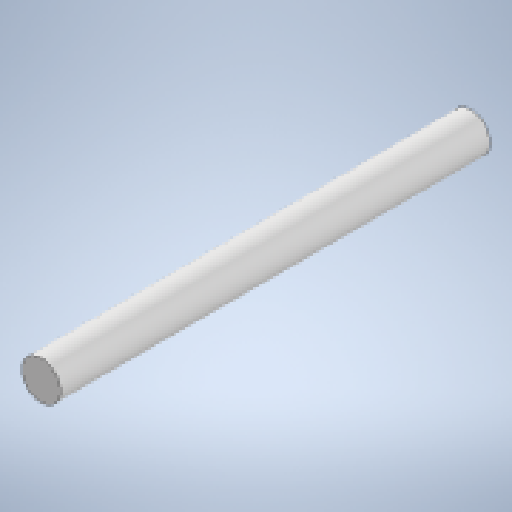
# Autodesk Inventor part: wał_2
Saved by Autodesk Inventor 2023 (Build 270158000, 158)
## iProperties
Created: 2023-03-11
Part Number: wał_2
Material: Ogólny
Document SubType Name: Modeling
Designer: Kamil
Density: 1 g/cm^3
Appearance: Domyślna
Author: Kamil
Autodesk Inventor part; units mm, degrees
ref_plane "YZ Plane" through (0, 0, 0) normal (1, 0, 0) x (0, 1, 0)
ref_plane "XZ Plane" through (0, 0, 0) normal (0, 1, 0) x (-1, 0, 0)
ref_plane "XY Plane" through (0, 0, 0) normal (0, 0, 1) x (1, 0, 0)
sketch "Szkic1" plane through (0, 0, 0) normal (0, 0, 1) x (1, 0, 0)
  circle A0 centre (-2.912, -2.7423) radius 5.3 projected
  circle A1 centre (-2.912, -2.7423) radius 5
  point P0 (0, 0)
  dimension "d0" = 10
  constraints: 1 centre point, 1 coincident
  measures "d0" diameter of A1
extrude "Wyciągnięcie proste1" add sketch "Szkic1" along normal blind 120 contours A1
move faces "Przesuń1" translate (0, 0, 5) faces at (-3.1129, -4.3968, 0)
move faces "Przesuń2" translate (0, 0, -4) faces at (-4.5787, -2.7423, 120)
